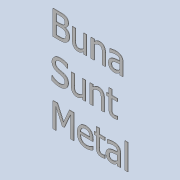
# Autodesk Inventor part: Orange
Saved by Autodesk Inventor 2020 (Build 240168000, 168)
## iProperties
Created: 2021-04-30
Part Number: Orange
Material: Generic
Document SubType Name: Modeling
Designer: Iulian Bors
Density: 1 g/cm^3
Appearance: Default
Author: Iulian Bors
Autodesk Inventor part; units mm, degrees
ref_plane "YZ Plane" through (0, 0, 0) normal (1, 0, 0) x (0, 1, 0)
ref_plane "XZ Plane" through (0, 0, 0) normal (0, 1, 0) x (-1, 0, 0)
ref_plane "XY Plane" through (0, 0, 0) normal (0, 0, 1) x (1, 0, 0)
sketch "Sketch1" plane through (0, 0, 0) normal (0, 0, 1) x (1, 0, 0)
  line L0 (-148.5, 210) -> (148.5, 210) construction
  line L1 (148.5, 210) -> (148.5, -210) construction
  line L2 (148.5, -210) -> (-148.5, -210) construction
  line L3 (-148.5, -210) -> (-148.5, 210) construction
  line L4 (-59.6293, 105.4874) -> (22.3804, 105.4874) construction
  line L5 (22.3804, 105.4874) -> (22.3804, -2.3631) construction
  line L6 (22.3804, -2.3631) -> (-59.6293, -2.3631) construction
  line L7 (-59.6293, -2.3631) -> (-59.6293, 105.4874) construction
  spline S0 degree 2 poles (-28.4462, 77.7726) (-28.4462, 74.7905) (-30.7152, 70.22) (-32.5953, 68.7289) knots 0 0 0 1 2 2 2
  spline S1 degree 2 poles (-32.5953, 68.7289) (-34.8643, 66.9785) (-40.0183, 65.4874) (-44.1026, 65.4874) knots 0 0 0 1 2 2 2
  line L8 (-44.1026, 65.4874) -> (-55.5775, 65.4874)
  line L9 (-55.5775, 65.4874) -> (-55.5775, 105.4874)
  line L10 (-55.5775, 105.4874) -> (-44.9778, 105.4874)
  spline S2 degree 2 poles (-44.9778, 105.4874) (-40.699, 105.4874) (-36.4203, 104.9363) (-34.4754, 103.8666) knots 0 0 0 1 2 2 2
  spline S3 degree 2 poles (-34.4754, 103.8666) (-32.3036, 102.7321) (-30.3263, 99.0044) (-30.3263, 96.476) knots 0 0 0 1 2 2 2
  spline S4 degree 2 poles (-30.3263, 96.476) (-30.3263, 93.6559) (-33.3084, 89.1827) (-35.934, 87.9185) knots 0 0 0 1 2 2 2
  line L11 (-35.934, 87.9185) -> (-35.934, 87.724)
  spline S5 degree 2 poles (-35.934, 87.724) (-32.3684, 86.7516) (-28.4462, 81.5976) (-28.4462, 77.7726) knots 0 0 0 1 2 2 2
  spline S6 degree 2 poles (-33.9891, 77.5457) (-33.9891, 79.8148) (-35.2857, 82.7321) (-37.2306, 83.7694) knots 0 0 0 1 2 2 2
  spline S7 degree 2 poles (-37.2306, 83.7694) (-38.4948, 84.4177) (-41.477, 84.8067) (-44.2323, 84.8067) knots 0 0 0 1 2 2 2
  line L12 (-44.2323, 84.8067) -> (-50.2614, 84.8067)
  line L13 (-50.2614, 84.8067) -> (-50.2614, 70.0255)
  line L14 (-50.2614, 70.0255) -> (-45.9502, 70.0255)
  spline S8 degree 2 poles (-45.9502, 70.0255) (-42.4494, 70.0255) (-38.43, 70.6738) (-36.8741, 71.711) knots 0 0 0 1 2 2 2
  spline S9 degree 2 poles (-36.8741, 71.711) (-35.383, 72.7807) (-33.9891, 75.4388) (-33.9891, 77.5457) knots 0 0 0 1 2 2 2
  spline S10 degree 2 poles (-35.8692, 95.7305) (-35.8692, 97.1567) (-36.8417, 99.2961) (-37.9113, 99.912) knots 0 0 0 1 2 2 2
  spline S11 degree 2 poles (-37.9113, 99.912) (-39.2079, 100.6251) (-42.3522, 100.9493) (-45.1723, 100.9493) knots 0 0 0 1 2 2 2
  line L15 (-45.1723, 100.9493) -> (-50.2614, 100.9493)
  line L16 (-50.2614, 100.9493) -> (-50.2614, 89.2475)
  line L17 (-50.2614, 89.2475) -> (-44.2323, 89.2475)
  spline S12 degree 2 poles (-44.2323, 89.2475) (-41.7363, 89.2475) (-39.37, 89.7661) (-38.1058, 90.5765) knots 0 0 0 1 2 2 2
  spline S13 degree 2 poles (-38.1058, 90.5765) (-36.8741, 91.3545) (-35.8692, 93.8504) (-35.8692, 95.7305) knots 0 0 0 1 2 2 2
  line L18 (-0.2128, 65.4874) -> (-5.2695, 65.4874)
  line L19 (-5.2695, 65.4874) -> (-5.2695, 68.7937)
  spline S14 degree 2 poles (-5.2695, 68.7937) (-7.6034, 66.7516) (-11.7849, 64.6446) (-14.3781, 64.6446) knots 0 0 0 1 2 2 2
  spline S15 degree 2 poles (-14.3781, 64.6446) (-16.323, 64.6446) (-19.7914, 65.9412) (-21.0556, 67.335) knots 0 0 0 1 2 2 2
  spline S16 degree 2 poles (-21.0556, 67.335) (-22.3522, 68.7289) (-23.7784, 72.9752) (-23.7784, 76.0222) knots 0 0 0 1 2 2 2
  line L20 (-23.7784, 76.0222) -> (-23.7784, 95.5036)
  line L21 (-23.7784, 95.5036) -> (-18.7217, 95.5036)
  line L22 (-18.7217, 95.5036) -> (-18.7217, 78.3885)
  spline S17 degree 2 poles (-18.7217, 78.3885) (-18.7217, 75.9898) (-18.3652, 72.8456) (-17.7493, 71.6786) knots 0 0 0 1 2 2 2
  spline S18 degree 2 poles (-17.7493, 71.6786) (-17.1334, 70.5117) (-15.0264, 69.442) (-13.0491, 69.442) knots 0 0 0 1 2 2 2
  spline S19 degree 2 poles (-13.0491, 69.442) (-11.2015, 69.442) (-7.0199, 71.549) (-5.2695, 73.0725) knots 0 0 0 1 2 2 2
  line L23 (-5.2695, 73.0725) -> (-5.2695, 95.5036)
  line L24 (-5.2695, 95.5036) -> (-0.2128, 95.5036)
  line L25 (-0.2128, 95.5036) -> (-0.2128, 65.4874)
  line L26 (30.6786, 65.4874) -> (25.6219, 65.4874)
  line L27 (25.6219, 65.4874) -> (25.6219, 82.6024)
  spline S20 degree 2 poles (25.6219, 82.6024) (25.6219, 84.677) (25.2329, 88.2426) (24.6494, 89.3123) knots 0 0 0 1 2 2 2
  spline S21 degree 2 poles (24.6494, 89.3123) (24.0335, 90.4469) (21.8293, 91.549) (19.9493, 91.549) knots 0 0 0 1 2 2 2
  spline S22 degree 2 poles (19.9493, 91.549) (18.0692, 91.549) (14.0822, 89.5392) (12.1697, 87.9185) knots 0 0 0 1 2 2 2
  line L28 (12.1697, 87.9185) -> (12.1697, 65.4874)
  line L29 (12.1697, 65.4874) -> (7.113, 65.4874)
  line L30 (7.113, 65.4874) -> (7.113, 95.5036)
  line L31 (7.113, 95.5036) -> (12.1697, 95.5036)
  line L32 (12.1697, 95.5036) -> (12.1697, 92.1648)
  spline S23 degree 2 poles (12.1697, 92.1648) (14.4387, 94.207) (18.8147, 96.3464) (21.2783, 96.3464) knots 0 0 0 1 2 2 2
  spline S24 degree 2 poles (21.2783, 96.3464) (25.6867, 96.3464) (30.6786, 90.5117) (30.6786, 84.9687) knots 0 0 0 1 2 2 2
  line L33 (30.6786, 84.9687) -> (30.6786, 65.4874)
  spline S25 degree 2 poles (54.5036, 68.664) (53.8877, 68.2102) (51.8131, 66.5895) (50.8407, 66.1033) knots 0 0 0 1 2 2 2
  spline S26 degree 2 poles (50.8407, 66.1033) (49.5117, 65.3901) (47.0157, 64.6446) (44.7467, 64.6446) knots 0 0 0 1 2 2 2
  spline S27 degree 2 poles (44.7467, 64.6446) (42.899, 64.6446) (39.5603, 66.0384) (38.2961, 67.3026) knots 0 0 0 1 2 2 2
  spline S28 degree 2 poles (38.2961, 67.3026) (37.0968, 68.5344) (35.6381, 72.1648) (35.6381, 74.1746) knots 0 0 0 1 2 2 2
  spline S29 degree 2 poles (35.6381, 74.1746) (35.6381, 77.2864) (38.2637, 81.6948) (41.1162, 82.959) knots 0 0 0 1 2 2 2
  spline S30 degree 2 poles (41.1162, 82.959) (43.6446, 84.1259) (50.5165, 85.0012) (54.5036, 85.2281) knots 0 0 0 1 2 2 2
  line L34 (54.5036, 85.2281) -> (54.5036, 86.2005)
  spline S31 degree 2 poles (54.5036, 86.2005) (54.5036, 87.9509) (53.4339, 90.1227) (52.4614, 90.7386) knots 0 0 0 1 2 2 2
  spline S32 degree 2 poles (52.4614, 90.7386) (51.489, 91.3545) (48.7013, 91.7435) (47.2102, 91.7435) knots 0 0 0 1 2 2 2
  spline S33 degree 2 poles (47.2102, 91.7435) (45.4598, 91.7435) (40.7272, 90.7062) (38.3609, 89.7013) knots 0 0 0 1 2 2 2
  line L35 (38.3609, 89.7013) -> (38.0692, 89.7013)
  line L36 (38.0692, 89.7013) -> (38.0692, 94.8553)
  spline S34 degree 2 poles (38.0692, 94.8553) (39.463, 95.2443) (44.6818, 96.2167) (47.2426, 96.2167) knots 0 0 0 1 2 2 2
  spline S35 degree 2 poles (47.2426, 96.2167) (50.3545, 96.2167) (54.6008, 95.2443) (56.2864, 93.9801) knots 0 0 0 1 2 2 2
  spline S36 degree 2 poles (56.2864, 93.9801) (57.9395, 92.7483) (59.5603, 88.8261) (59.5603, 86.006) knots 0 0 0 1 2 2 2
  line L37 (59.5603, 86.006) -> (59.5603, 65.4874)
  line L38 (59.5603, 65.4874) -> (54.5036, 65.4874)
  line L39 (54.5036, 65.4874) -> (54.5036, 68.664)
  line L40 (54.5036, 72.878) -> (54.5036, 81.2086)
  spline S37 degree 2 poles (54.5036, 81.2086) (52.6883, 81.0465) (47.2102, 80.4955) (45.4922, 79.9768) knots 0 0 0 1 2 2 2
  spline S38 degree 2 poles (45.4922, 79.9768) (43.4825, 79.361) (40.8569, 76.8002) (40.8569, 74.5311) knots 0 0 0 1 2 2 2
  spline S39 degree 2 poles (40.8569, 74.5311) (40.8569, 71.9379) (43.7742, 69.3123) (46.5619, 69.3123) knots 0 0 0 1 2 2 2
  spline S40 degree 2 poles (46.5619, 69.3123) (48.9282, 69.3123) (52.818, 71.3545) (54.5036, 72.878) knots 0 0 0 1 2 2 2
  spline S41 degree 2 poles (-44.4267, -1.0847) (-48.7703, -1.0847) (-54.8643, 0.7305) (-57.5548, 2.0271) knots 0 0 0 1 2 2 2
  line L41 (-57.5548, 2.0271) -> (-57.5548, 8.7046)
  line L42 (-57.5548, 8.7046) -> (-57.1658, 8.7046)
  spline S42 degree 2 poles (-57.1658, 8.7046) (-54.5402, 6.2411) (-47.8951, 3.5182) (-44.8157, 3.5182) knots 0 0 0 1 2 2 2
  spline S43 degree 2 poles (-44.8157, 3.5182) (-40.4073, 3.5182) (-35.9016, 7.1811) (-35.9016, 10.1957) knots 0 0 0 1 2 2 2
  spline S44 degree 2 poles (-35.9016, 10.1957) (-35.9016, 12.5944) (-38.2679, 15.5766) (-40.8287, 16.3221) knots 0 0 0 1 2 2 2
  spline S45 degree 2 poles (-40.8287, 16.3221) (-42.6763, 16.8407) (-45.7558, 17.5539) (-48.0572, 18.1373) knots 0 0 0 1 2 2 2
  spline S46 degree 2 poles (-48.0572, 18.1373) (-50.1318, 18.6884) (-53.4057, 20.3416) (-54.6699, 21.6706) knots 0 0 0 1 2 2 2
  spline S47 degree 2 poles (-54.6699, 21.6706) (-55.9016, 22.9996) (-57.263, 26.5652) (-57.263, 28.8991) knots 0 0 0 1 2 2 2
  spline S48 degree 2 poles (-57.263, 28.8991) (-57.263, 33.7613) (-49.678, 40.3416) (-43.8109, 40.3416) knots 0 0 0 1 2 2 2
  spline S49 degree 2 poles (-43.8109, 40.3416) (-40.4397, 40.3416) (-34.4754, 39.0125) (-31.9146, 37.7484) knots 0 0 0 1 2 2 2
  line L43 (-31.9146, 37.7484) -> (-31.9146, 31.395)
  line L44 (-31.9146, 31.395) -> (-32.3036, 31.395)
  spline S50 degree 2 poles (-32.3036, 31.395) (-34.216, 33.1454) (-40.1804, 35.7386) (-43.4543, 35.7386) knots 0 0 0 1 2 2 2
  spline S51 degree 2 poles (-43.4543, 35.7386) (-47.1496, 35.7386) (-51.7201, 32.2702) (-51.7201, 29.4501) knots 0 0 0 1 2 2 2
  spline S52 degree 2 poles (-51.7201, 29.4501) (-51.7201, 26.9218) (-49.0297, 23.9072) (-46.5013, 23.2265) knots 0 0 0 1 2 2 2
  spline S53 degree 2 poles (-46.5013, 23.2265) (-44.8157, 22.7727) (-39.9211, 21.6057) (-38.3003, 21.1195) knots 0 0 0 1 2 2 2
  spline S54 degree 2 poles (-38.3003, 21.1195) (-34.1836, 19.8553) (-30.3587, 14.7662) (-30.3587, 11.0385) knots 0 0 0 1 2 2 2
  spline S55 degree 2 poles (-30.3587, 11.0385) (-30.3587, 8.6722) (-32.2712, 4.1341) (-33.9891, 2.5458) knots 0 0 0 1 2 2 2
  spline S56 degree 2 poles (-33.9891, 2.5458) (-35.9016, 0.7954) (-40.7639, -1.0847) (-44.4267, -1.0847) knots 0 0 0 1 2 2 2
  line L45 (-1.9956, -0.3716) -> (-7.0524, -0.3716)
  line L46 (-7.0524, -0.3716) -> (-7.0524, 2.9347)
  spline S57 degree 2 poles (-7.0524, 2.9347) (-9.3862, 0.8926) (-13.5677, -1.2144) (-16.1609, -1.2144) knots 0 0 0 1 2 2 2
  spline S58 degree 2 poles (-16.1609, -1.2144) (-18.1058, -1.2144) (-21.5742, 0.0822) (-22.8384, 1.4761) knots 0 0 0 1 2 2 2
  spline S59 degree 2 poles (-22.8384, 1.4761) (-24.135, 2.8699) (-25.5613, 7.1163) (-25.5613, 10.1633) knots 0 0 0 1 2 2 2
  line L47 (-25.5613, 10.1633) -> (-25.5613, 29.6446)
  line L48 (-25.5613, 29.6446) -> (-20.5045, 29.6446)
  line L49 (-20.5045, 29.6446) -> (-20.5045, 12.5296)
  spline S60 degree 2 poles (-20.5045, 12.5296) (-20.5045, 10.1309) (-20.148, 6.9866) (-19.5321, 5.8197) knots 0 0 0 1 2 2 2
  spline S61 degree 2 poles (-19.5321, 5.8197) (-18.9162, 4.6527) (-16.8092, 3.583) (-14.8319, 3.583) knots 0 0 0 1 2 2 2
  spline S62 degree 2 poles (-14.8319, 3.583) (-12.9843, 3.583) (-8.8028, 5.69) (-7.0524, 7.2135) knots 0 0 0 1 2 2 2
  line L50 (-7.0524, 7.2135) -> (-7.0524, 29.6446)
  line L51 (-7.0524, 29.6446) -> (-1.9956, 29.6446)
  line L52 (-1.9956, 29.6446) -> (-1.9956, -0.3716)
  line L53 (28.8958, -0.3716) -> (23.8391, -0.3716)
  line L54 (23.8391, -0.3716) -> (23.8391, 16.7435)
  spline S63 degree 2 poles (23.8391, 16.7435) (23.8391, 18.8181) (23.4501, 22.3837) (22.8666, 23.4534) knots 0 0 0 1 2 2 2
  spline S64 degree 2 poles (22.8666, 23.4534) (22.2507, 24.5879) (20.0465, 25.69) (18.1664, 25.69) knots 0 0 0 1 2 2 2
  spline S65 degree 2 poles (18.1664, 25.69) (16.2864, 25.69) (12.2994, 23.6803) (10.3869, 22.0595) knots 0 0 0 1 2 2 2
  line L55 (10.3869, 22.0595) -> (10.3869, -0.3716)
  line L56 (10.3869, -0.3716) -> (5.3301, -0.3716)
  line L57 (5.3301, -0.3716) -> (5.3301, 29.6446)
  line L58 (5.3301, 29.6446) -> (10.3869, 29.6446)
  line L59 (10.3869, 29.6446) -> (10.3869, 26.3059)
  spline S66 degree 2 poles (10.3869, 26.3059) (12.6559, 28.348) (17.0319, 30.4874) (19.4955, 30.4874) knots 0 0 0 1 2 2 2
  spline S67 degree 2 poles (19.4955, 30.4874) (23.9039, 30.4874) (28.8958, 24.6527) (28.8958, 19.1098) knots 0 0 0 1 2 2 2
  line L60 (28.8958, 19.1098) -> (28.8958, -0.3716)
  spline S68 degree 2 poles (45.0708, -0.955) (40.9541, -0.955) (36.3188, 3.7451) (36.3188, 8.8343) knots 0 0 0 1 2 2 2
  line L61 (36.3188, 8.8343) -> (36.3188, 25.4631)
  line L62 (36.3188, 25.4631) -> (32.9152, 25.4631)
  line L63 (32.9152, 25.4631) -> (32.9152, 29.6446)
  line L64 (32.9152, 29.6446) -> (36.3188, 29.6446)
  line L65 (36.3188, 29.6446) -> (36.3188, 38.267)
  line L66 (36.3188, 38.267) -> (41.3755, 38.267)
  line L67 (41.3755, 38.267) -> (41.3755, 29.6446)
  line L68 (41.3755, 29.6446) -> (50.6786, 29.6446)
  line L69 (50.6786, 29.6446) -> (50.6786, 25.4631)
  line L70 (50.6786, 25.4631) -> (41.3755, 25.4631)
  line L71 (41.3755, 25.4631) -> (41.3755, 11.1681)
  spline S69 degree 2 poles (41.3755, 11.1681) (41.3755, 8.8991) (41.5376, 6.4031) (42.0887, 5.3335) knots 0 0 0 1 2 2 2
  spline S70 degree 2 poles (42.0887, 5.3335) (42.5425, 4.3934) (44.5846, 3.4534) (46.335, 3.4534) knots 0 0 0 1 2 2 2
  spline S71 degree 2 poles (46.335, 3.4534) (47.5668, 3.4534) (49.8682, 4.1989) (50.3869, 4.4258) knots 0 0 0 1 2 2 2
  line L72 (50.3869, 4.4258) -> (50.6786, 4.4258)
  line L73 (50.6786, 4.4258) -> (50.6786, -0.1123)
  spline S72 degree 2 poles (50.6786, -0.1123) (49.2523, -0.5012) (46.335, -0.955) (45.0708, -0.955) knots 0 0 0 1 2 2 2
  line L74 (-21.2825, -66.2305) -> (-26.5985, -66.2305)
  line L75 (-26.5985, -66.2305) -> (-26.5985, -31.7735)
  line L76 (-26.5985, -31.7735) -> (-37.0361, -55.2094)
  line L77 (-37.0361, -55.2094) -> (-40.2776, -55.2094)
  line L78 (-40.2776, -55.2094) -> (-50.618, -31.7735)
  line L79 (-50.618, -31.7735) -> (-50.618, -66.2305)
  line L80 (-50.618, -66.2305) -> (-55.5775, -66.2305)
  line L81 (-55.5775, -66.2305) -> (-55.5775, -26.2305)
  line L82 (-55.5775, -26.2305) -> (-48.3165, -26.2305)
  line L83 (-48.3165, -26.2305) -> (-38.3327, -48.4996)
  line L84 (-38.3327, -48.4996) -> (-28.6731, -26.2305)
  line L85 (-28.6731, -26.2305) -> (-21.2825, -26.2305)
  line L86 (-21.2825, -26.2305) -> (-21.2825, -66.2305)
  spline S73 degree 2 poles (-0.537, -66.9112) (-7.7331, -66.9112) (-15.6423, -58.8399) (-15.6423, -51.3845) knots 0 0 0 1 2 2 2
  spline S74 degree 2 poles (-15.6423, -51.3845) (-15.6423, -44.0587) (-7.96, -35.3715) (-1.7687, -35.3715) knots 0 0 0 1 2 2 2
  spline S75 degree 2 poles (-1.7687, -35.3715) (1.019, -35.3715) (5.3301, -36.9923) (6.9185, -38.7103) knots 0 0 0 1 2 2 2
  spline S76 degree 2 poles (6.9185, -38.7103) (8.5392, -40.4282) (10.2572, -45.3877) (10.2572, -48.9858) knots 0 0 0 1 2 2 2
  line L87 (10.2572, -48.9858) -> (10.2572, -51.7411)
  line L88 (10.2572, -51.7411) -> (-10.5207, -51.7411)
  spline S77 degree 2 poles (-10.5207, -51.7411) (-10.5207, -56.9599) (-5.2695, -62.5028) (-0.6018, -62.5028) knots 0 0 0 1 2 2 2
  spline S78 degree 2 poles (-0.6018, -62.5028) (1.0514, -62.5028) (4.2605, -61.7573) (5.557, -61.1738) knots 0 0 0 1 2 2 2
  spline S79 degree 2 poles (5.557, -61.1738) (6.9185, -60.5255) (8.7985, -59.391) (9.4144, -58.8723) knots 0 0 0 1 2 2 2
  line L89 (9.4144, -58.8723) -> (9.7062, -58.8723)
  line L90 (9.7062, -58.8723) -> (9.7062, -64.3829)
  spline S80 degree 2 poles (9.7062, -64.3829) (8.831, -64.7394) (6.1729, -65.7767) (5.1357, -66.0684) knots 0 0 0 1 2 2 2
  spline S81 degree 2 poles (5.1357, -66.0684) (3.677, -66.4898) (1.2783, -66.9112) (-0.537, -66.9112) knots 0 0 0 1 2 2 2
  spline S82 degree 2 poles (5.3301, -47.8837) (5.2653, -45.8415) (4.4225, -42.8594) (3.6122, -41.8545) knots 0 0 0 1 2 2 2
  spline S83 degree 2 poles (3.6122, -41.8545) (2.737, -40.72) (-0.0183, -39.5206) (-2.0605, -39.5206) knots 0 0 0 1 2 2 2
  spline S84 degree 2 poles (-2.0605, -39.5206) (-4.0702, -39.5206) (-6.8903, -40.72) (-8.0572, -41.8869) knots 0 0 0 1 2 2 2
  spline S85 degree 2 poles (-8.0572, -41.8869) (-9.1917, -43.0863) (-10.3587, -45.9712) (-10.5207, -47.8837) knots 0 0 0 1 2 2 2
  line L91 (-10.5207, -47.8837) -> (5.3301, -47.8837)
  spline S86 degree 2 poles (24.4549, -66.814) (20.3382, -66.814) (15.7029, -62.1138) (15.7029, -57.0247) knots 0 0 0 1 2 2 2
  line L92 (15.7029, -57.0247) -> (15.7029, -40.3958)
  line L93 (15.7029, -40.3958) -> (12.2994, -40.3958)
  line L94 (12.2994, -40.3958) -> (12.2994, -36.2143)
  line L95 (12.2994, -36.2143) -> (15.7029, -36.2143)
  line L96 (15.7029, -36.2143) -> (15.7029, -27.5919)
  line L97 (15.7029, -27.5919) -> (20.7596, -27.5919)
  line L98 (20.7596, -27.5919) -> (20.7596, -36.2143)
  line L99 (20.7596, -36.2143) -> (30.0627, -36.2143)
  line L100 (30.0627, -36.2143) -> (30.0627, -40.3958)
  line L101 (30.0627, -40.3958) -> (20.7596, -40.3958)
  line L102 (20.7596, -40.3958) -> (20.7596, -54.6908)
  spline S87 degree 2 poles (20.7596, -54.6908) (20.7596, -56.9599) (20.9217, -59.4558) (21.4728, -60.5255) knots 0 0 0 1 2 2 2
  spline S88 degree 2 poles (21.4728, -60.5255) (21.9266, -61.4655) (23.9687, -62.4056) (25.7191, -62.4056) knots 0 0 0 1 2 2 2
  spline S89 degree 2 poles (25.7191, -62.4056) (26.9509, -62.4056) (29.2523, -61.66) (29.771, -61.4331) knots 0 0 0 1 2 2 2
  line L103 (29.771, -61.4331) -> (30.0627, -61.4331)
  line L104 (30.0627, -61.4331) -> (30.0627, -65.9712)
  spline S90 degree 2 poles (30.0627, -65.9712) (28.6365, -66.3602) (25.7191, -66.814) (24.4549, -66.814) knots 0 0 0 1 2 2 2
  spline S91 degree 2 poles (50.5165, -63.0539) (49.9006, -63.5077) (47.8261, -65.1284) (46.8536, -65.6146) knots 0 0 0 1 2 2 2
  spline S92 degree 2 poles (46.8536, -65.6146) (45.5246, -66.3278) (43.0287, -67.0733) (40.7596, -67.0733) knots 0 0 0 1 2 2 2
  spline S93 degree 2 poles (40.7596, -67.0733) (38.912, -67.0733) (35.5733, -65.6795) (34.3091, -64.4153) knots 0 0 0 1 2 2 2
  spline S94 degree 2 poles (34.3091, -64.4153) (33.1097, -63.1835) (31.6511, -59.553) (31.6511, -57.5433) knots 0 0 0 1 2 2 2
  spline S95 degree 2 poles (31.6511, -57.5433) (31.6511, -54.4315) (34.2767, -50.0231) (37.1292, -48.7589) knots 0 0 0 1 2 2 2
  spline S96 degree 2 poles (37.1292, -48.7589) (39.6575, -47.5919) (46.5295, -46.7167) (50.5165, -46.4898) knots 0 0 0 1 2 2 2
  line L105 (50.5165, -46.4898) -> (50.5165, -45.5174)
  spline S97 degree 2 poles (50.5165, -45.5174) (50.5165, -43.767) (49.4468, -41.5952) (48.4744, -40.9793) knots 0 0 0 1 2 2 2
  spline S98 degree 2 poles (48.4744, -40.9793) (47.5019, -40.3634) (44.7143, -39.9744) (43.2232, -39.9744) knots 0 0 0 1 2 2 2
  spline S99 degree 2 poles (43.2232, -39.9744) (41.4728, -39.9744) (36.7402, -41.0117) (34.3739, -42.0166) knots 0 0 0 1 2 2 2
  line L106 (34.3739, -42.0166) -> (34.0822, -42.0166)
  line L107 (34.0822, -42.0166) -> (34.0822, -36.8626)
  spline S100 degree 2 poles (34.0822, -36.8626) (35.476, -36.4736) (40.6948, -35.5012) (43.2556, -35.5012) knots 0 0 0 1 2 2 2
  spline S101 degree 2 poles (43.2556, -35.5012) (46.3674, -35.5012) (50.6138, -36.4736) (52.2994, -37.7378) knots 0 0 0 1 2 2 2
  spline S102 degree 2 poles (52.2994, -37.7378) (53.9525, -38.9696) (55.5733, -42.8918) (55.5733, -45.7119) knots 0 0 0 1 2 2 2
  line L108 (55.5733, -45.7119) -> (55.5733, -66.2305)
  line L109 (55.5733, -66.2305) -> (50.5165, -66.2305)
  line L110 (50.5165, -66.2305) -> (50.5165, -63.0539)
  line L111 (50.5165, -58.8399) -> (50.5165, -50.5093)
  spline S103 degree 2 poles (50.5165, -50.5093) (48.7013, -50.6714) (43.2232, -51.2224) (41.5052, -51.7411) knots 0 0 0 1 2 2 2
  spline S104 degree 2 poles (41.5052, -51.7411) (39.4955, -52.3569) (36.8699, -54.9177) (36.8699, -57.1868) knots 0 0 0 1 2 2 2
  spline S105 degree 2 poles (36.8699, -57.1868) (36.8699, -59.7799) (39.7872, -62.4056) (42.5749, -62.4056) knots 0 0 0 1 2 2 2
  spline S106 degree 2 poles (42.5749, -62.4056) (44.9412, -62.4056) (48.831, -60.3634) (50.5165, -58.8399) knots 0 0 0 1 2 2 2
  line L112 (67.8261, -66.2305) -> (62.7694, -66.2305)
  line L113 (62.7694, -66.2305) -> (62.7694, -24.4477)
  line L114 (62.7694, -24.4477) -> (67.8261, -24.4477)
  line L115 (67.8261, -24.4477) -> (67.8261, -66.2305)
  point P0 (0, 0)
  point P1 (0, 210)
  point P2 (-148.5, 0)
  dimension "d0" = 297
  dimension "d1" = 420
  constraints: 8 end point, 2 midpoint, 2 parallel, 1 horizontal, 1 horizontal alignment, 1 perpendicular, 1 vertical alignment, 2 other
  measures "d0" distance of L0.start L0.end
  measures "d1" distance of L2.end L0.start
extrude "Extrusion1" add sketch "Sketch1" along normal blind 0.8
body "Solid1"
